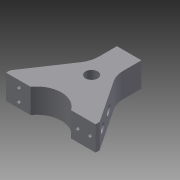
# Autodesk Inventor part: front leg
Saved by Autodesk Inventor 2013 (Build 170138000, 138)
## iProperties
Created: 2013-09-23
Part Number: front leg
Material: Generic
Document SubType Name: Modeling
Designer: Ian
Density: 1 g/cm^3
Author: Ian
Autodesk Inventor part; units mm, degrees
ref_plane "YZ Plane" through (0, 0, 0) normal (1, 0, 0) x (0, 1, 0)
ref_plane "XZ Plane" through (0, 0, 0) normal (0, 1, 0) x (-1, 0, 0)
ref_plane "XY Plane" through (0, 0, 0) normal (0, 0, 1) x (1, 0, 0)
sketch "Sketch1" plane through (0, 0, 0) normal (0, 1, 0) x (-1, 0, 0)
  line L0 (19.05, -18.5452) -> (19.05, -58.42)
  line L1 (19.05, -58.42) -> (0, -58.42)
  line L2 (19.05, -58.42) -> (19.05, -18.5452)
  line L3 (31.496, 63.5) -> (69.596, 63.5)
  arc A0 (0, 47.0625) -> (31.496, 63.5) centre (0, 85.4562) ccw
  line L4 (0, 85.4562) -> (0, -58.42) construction
  line L5 (69.596, 63.5) -> (69.596, 57.15)
  line L6 (69.596, 57.15) -> (19.05, -18.5452)
  line L7 (0, 0) -> (69.596, 0) construction
  line L8 (-19.05, -58.42) -> (0, -58.42)
  line L9 (-19.05, -58.42) -> (-19.05, -18.5452)
  line L10 (-31.496, 63.5) -> (-69.596, 63.5)
  arc A1 (-31.496, 63.5) -> (0, 47.0625) centre (0, 85.4562) ccw
  line L11 (-69.596, 63.5) -> (-69.596, 57.15)
  line L12 (-69.596, 57.15) -> (-19.05, -18.5452)
  dimension "d73" = 38.3937
  dimension "d74" = 57.15
  dimension "d75" = 18.5452
  dimension "d76" = 19.05
  dimension "d77" = 58.42
  dimension "d78" = 69.596
  dimension "d79" = 38.1
  dimension "d80" = 31.496
  dimension "d81" = 63.5
  dimension "d82" = 6.35
  dimension "d83" = 39.8748
  dimension "d84" = 47.0626
  dimension "d86" = 121.92
  dimension "d90" = 38.1
  constraints: 26 end point, 6 symmetric about line, 4 point on circle, 3 horizontal, 3 point on line, 2 centre point, 2 vertical, 1 coincident, 1 perpendicular, 1 other
  measures "d73" radius of A0
  measures "d74" distance of L7.end L5.end
  measures "d75" vertical distance of L7.end L0.start
  measures "d76" distance from line of L0.start L4
  measures "d77" vertical distance of L0.end L7.end
  measures "d78" distance from line of L3.end L4
  measures "d79" distance of L3.start L3.end
  measures "d80" distance from line of L3.start L4
  measures "d81" distance from line of L7 L3.start
  measures "d82" distance of L3.end L5.end
  measures "d83" distance of L0.start L0.end
  measures "d84" distance of L7.start A0.start
  measures "d86" vertical distance of L0.end L3.end
  measures "d90" distance of L9.start L0.end
extrude "Extrusion1" add sketch "Sketch1" along normal blind 38.1
hole "Hole1" at (0, 0, 0) direction (0, 1, 0) diameter 19.05 end through all
sketch "Sketch2" plane through (19.05, 0, -58.42) normal (0, 0, -1) x (-1, 0, 0)
  line L0 (38.1, 0) -> (88.646, 0) projected
  line L1 (88.646, 0) -> (88.646, 38.1) projected
  line L2 (38.1, 38.1) -> (88.646, 38.1) projected
  line L3 (38.1, 0) -> (38.1, 38.1) projected
  line L4 (-50.546, 0) -> (0, 0) projected
  line L5 (0, 0) -> (0, 38.1) projected
  line L6 (-50.546, 38.1) -> (0, 38.1) projected
  line L7 (-50.546, 0) -> (-50.546, 38.1) projected
  line L8 (88.646, 0) -> (50.546, 0) projected
  line L9 (50.546, 0) -> (50.546, 38.1) projected
  line L10 (88.646, 38.1) -> (50.546, 38.1) projected
  line L11 (88.646, 0) -> (88.646, 38.1) projected
  line L12 (69.596, 38.1) -> (69.596, 0) construction
  line L13 (-12.446, 0) -> (-12.446, 38.1) construction
  line L14 (-50.546, 19.05) -> (-12.446, 19.05) construction
  point P0 (19.05, 0)
  point P1 (-41.021, 19.05)
  point P2 (-21.971, 19.05)
  point P3 (69.596, 28.575)
  point P4 (69.596, 9.525)
  dimension "d92" = 38.1
  dimension "d93" = 9.525
  dimension "d94" = 9.525
  dimension "d95" = 9.525
  dimension "d96" = 9.525
  dimension "d97" = 38.1
  constraints: 4 end point, 4 midpoint, 4 point on line, 1 perpendicular
  measures "d92" distance of L9.end L1.end
  measures "d93" distance from line of L2 point (69.596, 28.575)
  measures "d94" distance from line of L0 point (69.596, 9.525)
  measures "d95" distance from line of L13 point (-21.971, 19.05)
  measures "d96" distance from line of L7 point (-41.021, 19.05)
  measures "d97" distance between parallel lines of L7 L13
hole "Hole2" at (60.071, 19.05, -58.42) at (41.021, 19.05, -58.42) at (-50.546, 28.575, -58.42) at (-50.546, 9.525, -58.42) direction (0, 0, 1) diameter 6.5278 depth 121.92 counterbore diameter 11.1252 counterbore depth 110.49 clearance for "Socket Head Cap Screw" size "1/4" standard "Ansi Unified Screw Threads"
fillet "Fillet1" radius 38.1 2 edges at (19.05, 19.05, -18.5452) (-19.05, 19.05, -18.5452)
equation "\"d94\" = d93"
equation "\"d95\" = d93"
equation "\"d96\" = d95"
body "Solid1"
